Autodesk Fusion 360 part; units mm, degrees
(part 12 of 18)
  arc A1395 (119.7972, -42.2017) -> (118.5972, -42.2017) centre (119.1972, -42.2017) ccw
  arc A1396 (119.7972, -42.2017) -> (118.5972, -42.2017) centre (119.1972, -42.2017) ccw
  arc A1397 (118.5972, -42.2017) -> (119.7972, -42.2017) centre (119.1972, -42.2017) ccw
  arc A1398 (118.5972, -42.2017) -> (119.7972, -42.2017) centre (119.1972, -42.2017) ccw
  arc A1399 (119.7972, -42.2017) -> (118.5972, -42.2017) centre (119.1972, -42.2017) ccw
  arc A1400 (116.2972, -44.4557) -> (115.0972, -44.4557) centre (115.6972, -44.4557) ccw
  arc A1401 (115.0972, -44.4557) -> (116.2972, -44.4557) centre (115.6972, -44.4557) ccw
  arc A1402 (116.2972, -44.4557) -> (115.0972, -44.4557) centre (115.6972, -44.4557) ccw
  arc A1403 (115.0972, -44.4557) -> (116.2972, -44.4557) centre (115.6972, -44.4557) ccw
  arc A1404 (116.2972, -44.4557) -> (115.0972, -44.4557) centre (115.6972, -44.4557) ccw
  arc A1405 (115.0972, -44.4557) -> (116.2972, -44.4557) centre (115.6972, -44.4557) ccw
  arc A1406 (100.7472, -23.1516) -> (99.5472, -23.1516) centre (100.1472, -23.1516) ccw
  arc A1407 (99.5472, -23.1516) -> (100.7472, -23.1516) centre (100.1472, -23.1516) ccw
  arc A1408 (100.7472, -23.1516) -> (99.5472, -23.1516) centre (100.1472, -23.1516) ccw
  arc A1409 (99.5472, -23.1516) -> (100.7472, -23.1516) centre (100.1472, -23.1516) ccw
  arc A1410 (99.5472, -23.1516) -> (100.7472, -23.1516) centre (100.1472, -23.1516) ccw
  arc A1411 (100.7472, -23.1516) -> (99.5472, -23.1516) centre (100.1472, -23.1516) ccw
  arc A1412 (97.2472, -25.4057) -> (96.0472, -25.4057) centre (96.6472, -25.4057) ccw
  arc A1413 (96.0472, -25.4057) -> (97.2472, -25.4057) centre (96.6472, -25.4057) ccw
  arc A1414 (97.2472, -25.4057) -> (96.0472, -25.4057) centre (96.6472, -25.4057) ccw
  arc A1415 (96.0472, -25.4057) -> (97.2472, -25.4057) centre (96.6472, -25.4057) ccw
  arc A1416 (97.2472, -25.4057) -> (96.0472, -25.4057) centre (96.6472, -25.4057) ccw
  arc A1417 (96.0472, -25.4057) -> (97.2472, -25.4057) centre (96.6472, -25.4057) ccw
  arc A1418 (100.7472, -42.2017) -> (99.5472, -42.2017) centre (100.1472, -42.2017) ccw
  arc A1419 (99.5472, -42.2017) -> (100.7472, -42.2017) centre (100.1472, -42.2017) ccw
  arc A1420 (100.7472, -42.2017) -> (99.5472, -42.2017) centre (100.1472, -42.2017) ccw
  arc A1421 (99.5472, -42.2017) -> (100.7472, -42.2017) centre (100.1472, -42.2017) ccw
  arc A1422 (100.7472, -42.2017) -> (99.5472, -42.2017) centre (100.1472, -42.2017) ccw
  arc A1423 (99.5472, -42.2017) -> (100.7472, -42.2017) centre (100.1472, -42.2017) ccw
  arc A1424 (97.2472, -44.4557) -> (96.0472, -44.4557) centre (96.6472, -44.4557) ccw
  arc A1425 (96.0472, -44.4557) -> (97.2472, -44.4557) centre (96.6472, -44.4557) ccw
  arc A1426 (96.0472, -44.4557) -> (97.2472, -44.4557) centre (96.6472, -44.4557) ccw
  arc A1427 (97.2472, -44.4557) -> (96.0472, -44.4557) centre (96.6472, -44.4557) ccw
  arc A1428 (96.0472, -44.4557) -> (97.2472, -44.4557) centre (96.6472, -44.4557) ccw
  arc A1429 (97.2472, -44.4557) -> (96.0472, -44.4557) centre (96.6472, -44.4557) ccw
  arc A1430 (100.7472, -80.3272) -> (99.5472, -80.3272) centre (100.1472, -80.3272) ccw
  arc A1431 (99.5472, -80.3272) -> (100.7472, -80.3272) centre (100.1472, -80.3272) ccw
  arc A1432 (100.7472, -80.3272) -> (99.5472, -80.3272) centre (100.1472, -80.3272) ccw
  arc A1433 (99.5472, -80.3272) -> (100.7472, -80.3272) centre (100.1472, -80.3272) ccw
  arc A1434 (99.5472, -80.3272) -> (100.7472, -80.3272) centre (100.1472, -80.3272) ccw
  arc A1435 (100.7472, -80.3272) -> (99.5472, -80.3272) centre (100.1472, -80.3272) ccw
  arc A1436 (97.2472, -82.5812) -> (96.0472, -82.5812) centre (96.6472, -82.5812) ccw
  arc A1437 (96.0472, -82.5812) -> (97.2472, -82.5812) centre (96.6472, -82.5812) ccw
  arc A1438 (97.2472, -82.5812) -> (96.0472, -82.5812) centre (96.6472, -82.5812) ccw
  arc A1439 (96.0472, -82.5812) -> (97.2472, -82.5812) centre (96.6472, -82.5812) ccw
  arc A1440 (97.2472, -82.5812) -> (96.0472, -82.5812) centre (96.6472, -82.5812) ccw
  arc A1441 (96.0472, -82.5812) -> (97.2472, -82.5812) centre (96.6472, -82.5812) ccw
  arc A1442 (99.5472, -61.2644) -> (100.7472, -61.2644) centre (100.1472, -61.2644) ccw
  arc A1443 (100.7472, -61.2644) -> (99.5472, -61.2644) centre (100.1472, -61.2644) ccw
  arc A1444 (100.7472, -61.2644) -> (99.5472, -61.2644) centre (100.1472, -61.2644) ccw
  arc A1445 (99.5472, -61.2644) -> (100.7472, -61.2644) centre (100.1472, -61.2644) ccw
  arc A1446 (99.5472, -61.2644) -> (100.7472, -61.2644) centre (100.1472, -61.2644) ccw
  arc A1447 (100.7472, -61.2644) -> (99.5472, -61.2644) centre (100.1472, -61.2644) ccw
  arc A1448 (96.0472, -63.5184) -> (97.2472, -63.5184) centre (96.6472, -63.5184) ccw
  arc A1449 (97.2472, -63.5184) -> (96.0472, -63.5184) centre (96.6472, -63.5184) ccw
  arc A1450 (97.2472, -63.5184) -> (96.0472, -63.5184) centre (96.6472, -63.5184) ccw
  arc A1451 (96.0472, -63.5184) -> (97.2472, -63.5184) centre (96.6472, -63.5184) ccw
  arc A1452 (97.2472, -63.5184) -> (96.0472, -63.5184) centre (96.6472, -63.5184) ccw
  arc A1453 (96.0472, -63.5184) -> (97.2472, -63.5184) centre (96.6472, -63.5184) ccw
  arc A1454 (194.7974, -80.3272) -> (195.9974, -80.3272) centre (195.3974, -80.3272) ccw
  arc A1455 (195.9974, -80.3272) -> (194.7974, -80.3272) centre (195.3974, -80.3272) ccw
  arc A1456 (194.7974, -80.3272) -> (195.9974, -80.3272) centre (195.3974, -80.3272) ccw
  arc A1457 (195.9974, -80.3272) -> (194.7974, -80.3272) centre (195.3974, -80.3272) ccw
  arc A1458 (194.7974, -80.3272) -> (195.9974, -80.3272) centre (195.3974, -80.3272) ccw
  arc A1459 (195.9974, -80.3272) -> (194.7974, -80.3272) centre (195.3974, -80.3272) ccw
  arc A1460 (192.4974, -82.5812) -> (191.2974, -82.5812) centre (191.8974, -82.5812) ccw
  arc A1461 (191.2974, -82.5812) -> (192.4974, -82.5812) centre (191.8974, -82.5812) ccw
  arc A1462 (191.2974, -82.5812) -> (192.4974, -82.5812) centre (191.8974, -82.5812) ccw
  arc A1463 (192.4974, -82.5812) -> (191.2974, -82.5812) centre (191.8974, -82.5812) ccw
  arc A1464 (192.4974, -82.5812) -> (191.2974, -82.5812) centre (191.8974, -82.5812) ccw
  arc A1465 (191.2974, -82.5812) -> (192.4974, -82.5812) centre (191.8974, -82.5812) ccw
  arc A1466 (195.9974, -23.1516) -> (194.7974, -23.1516) centre (195.3974, -23.1516) ccw
  arc A1467 (194.7974, -23.1516) -> (195.9974, -23.1516) centre (195.3974, -23.1516) ccw
  arc A1468 (194.7974, -23.1516) -> (195.9974, -23.1516) centre (195.3974, -23.1516) ccw
  arc A1469 (195.9974, -23.1516) -> (194.7974, -23.1516) centre (195.3974, -23.1516) ccw
  arc A1470 (195.9974, -23.1516) -> (194.7974, -23.1516) centre (195.3974, -23.1516) ccw
  arc A1471 (194.7974, -23.1516) -> (195.9974, -23.1516) centre (195.3974, -23.1516) ccw
  arc A1472 (192.4974, -25.4057) -> (191.2974, -25.4057) centre (191.8974, -25.4057) ccw
  arc A1473 (191.2974, -25.4057) -> (192.4974, -25.4057) centre (191.8974, -25.4057) ccw
  arc A1474 (191.2974, -25.4057) -> (192.4974, -25.4057) centre (191.8974, -25.4057) ccw
  arc A1475 (192.4974, -25.4057) -> (191.2974, -25.4057) centre (191.8974, -25.4057) ccw
  arc A1476 (192.4974, -25.4057) -> (191.2974, -25.4057) centre (191.8974, -25.4057) ccw
  arc A1477 (191.2974, -25.4057) -> (192.4974, -25.4057) centre (191.8974, -25.4057) ccw
  arc A1478 (81.6972, -80.3272) -> (80.4972, -80.3272) centre (81.0972, -80.3272) ccw
  arc A1479 (80.4972, -80.3272) -> (81.6972, -80.3272) centre (81.0972, -80.3272) ccw
  arc A1480 (81.6972, -80.3272) -> (80.4972, -80.3272) centre (81.0972, -80.3272) ccw
  arc A1481 (80.4972, -80.3272) -> (81.6972, -80.3272) centre (81.0972, -80.3272) ccw
  arc A1482 (80.4972, -80.3272) -> (81.6972, -80.3272) centre (81.0972, -80.3272) ccw
  arc A1483 (81.6972, -80.3272) -> (80.4972, -80.3272) centre (81.0972, -80.3272) ccw
  arc A1484 (76.9972, -82.5812) -> (78.1972, -82.5812) centre (77.5972, -82.5812) ccw
  arc A1485 (78.1972, -82.5812) -> (76.9972, -82.5812) centre (77.5972, -82.5812) ccw
  arc A1486 (76.9972, -82.5812) -> (78.1972, -82.5812) centre (77.5972, -82.5812) ccw
  arc A1487 (78.1972, -82.5812) -> (76.9972, -82.5812) centre (77.5972, -82.5812) ccw
  arc A1488 (78.1972, -82.5812) -> (76.9972, -82.5812) centre (77.5972, -82.5812) ccw
  arc A1489 (76.9972, -82.5812) -> (78.1972, -82.5812) centre (77.5972, -82.5812) ccw
  arc A1490 (81.6972, -42.2017) -> (80.4972, -42.2017) centre (81.0972, -42.2017) ccw
  arc A1491 (80.4972, -42.2017) -> (81.6972, -42.2017) centre (81.0972, -42.2017) ccw
  arc A1492 (81.6972, -42.2017) -> (80.4972, -42.2017) centre (81.0972, -42.2017) ccw
  arc A1493 (80.4972, -42.2017) -> (81.6972, -42.2017) centre (81.0972, -42.2017) ccw
  arc A1494 (81.6972, -42.2017) -> (80.4972, -42.2017) centre (81.0972, -42.2017) ccw
  arc A1495 (80.4972, -42.2017) -> (81.6972, -42.2017) centre (81.0972, -42.2017) ccw
  arc A1496 (78.1972, -44.4557) -> (76.9972, -44.4557) centre (77.5972, -44.4557) ccw
  arc A1497 (76.9972, -44.4557) -> (78.1972, -44.4557) centre (77.5972, -44.4557) ccw
  arc A1498 (76.9972, -44.4557) -> (78.1972, -44.4557) centre (77.5972, -44.4557) ccw
  arc A1499 (78.1972, -44.4557) -> (76.9972, -44.4557) centre (77.5972, -44.4557) ccw
  arc A1500 (78.1972, -44.4557) -> (76.9972, -44.4557) centre (77.5972, -44.4557) ccw
  arc A1501 (76.9972, -44.4557) -> (78.1972, -44.4557) centre (77.5972, -44.4557) ccw
  arc A1502 (80.4972, -23.1516) -> (81.6972, -23.1516) centre (81.0972, -23.1516) ccw
  arc A1503 (81.6972, -23.1516) -> (80.4972, -23.1516) centre (81.0972, -23.1516) ccw
  arc A1504 (80.4972, -23.1516) -> (81.6972, -23.1516) centre (81.0972, -23.1516) ccw
  arc A1505 (81.6972, -23.1516) -> (80.4972, -23.1516) centre (81.0972, -23.1516) ccw
  arc A1506 (81.6972, -23.1516) -> (80.4972, -23.1516) centre (81.0972, -23.1516) ccw
  arc A1507 (80.4972, -23.1516) -> (81.6972, -23.1516) centre (81.0972, -23.1516) ccw
  arc A1508 (78.1972, -25.4057) -> (76.9972, -25.4057) centre (77.5972, -25.4057) ccw
  arc A1509 (76.9972, -25.4057) -> (78.1972, -25.4057) centre (77.5972, -25.4057) ccw
  arc A1510 (76.9972, -25.4057) -> (78.1972, -25.4057) centre (77.5972, -25.4057) ccw
  arc A1511 (78.1972, -25.4057) -> (76.9972, -25.4057) centre (77.5972, -25.4057) ccw
  arc A1512 (76.9972, -25.4057) -> (78.1972, -25.4057) centre (77.5972, -25.4057) ccw
  arc A1513 (78.1972, -25.4057) -> (76.9972, -25.4057) centre (77.5972, -25.4057) ccw
  arc A1514 (80.4972, -61.2644) -> (81.6972, -61.2644) centre (81.0972, -61.2644) ccw
  arc A1515 (81.6972, -61.2644) -> (80.4972, -61.2644) centre (81.0972, -61.2644) ccw
  arc A1516 (81.6972, -61.2644) -> (80.4972, -61.2644) centre (81.0972, -61.2644) ccw
  arc A1517 (80.4972, -61.2644) -> (81.6972, -61.2644) centre (81.0972, -61.2644) ccw
  arc A1518 (81.6972, -61.2644) -> (80.4972, -61.2644) centre (81.0972, -61.2644) ccw
  arc A1519 (80.4972, -61.2644) -> (81.6972, -61.2644) centre (81.0972, -61.2644) ccw
  arc A1520 (76.9972, -63.5184) -> (78.1972, -63.5184) centre (77.5972, -63.5184) ccw
  arc A1521 (78.1972, -63.5184) -> (76.9972, -63.5184) centre (77.5972, -63.5184) ccw
  arc A1522 (78.1972, -63.5184) -> (76.9972, -63.5184) centre (77.5972, -63.5184) ccw
  arc A1523 (76.9972, -63.5184) -> (78.1972, -63.5184) centre (77.5972, -63.5184) ccw
  arc A1524 (78.1972, -63.5184) -> (76.9972, -63.5184) centre (77.5972, -63.5184) ccw
  arc A1525 (76.9972, -63.5184) -> (78.1972, -63.5184) centre (77.5972, -63.5184) ccw
  arc A1526 (61.4471, -80.3272) -> (62.6471, -80.3272) centre (62.0471, -80.3272) ccw
  arc A1527 (62.6471, -80.3272) -> (61.4471, -80.3272) centre (62.0471, -80.3272) ccw
  arc A1528 (61.4471, -80.3272) -> (62.6471, -80.3272) centre (62.0471, -80.3272) ccw
  arc A1529 (62.6471, -80.3272) -> (61.4471, -80.3272) centre (62.0471, -80.3272) ccw
  arc A1530 (61.4471, -80.3272) -> (62.6471, -80.3272) centre (62.0471, -80.3272) ccw
  arc A1531 (62.6471, -80.3272) -> (61.4471, -80.3272) centre (62.0471, -80.3272) ccw
  arc A1532 (59.1471, -82.5812) -> (57.9471, -82.5812) centre (58.5471, -82.5812) ccw
  arc A1533 (57.9471, -82.5812) -> (59.1471, -82.5812) centre (58.5471, -82.5812) ccw
  arc A1534 (57.9471, -82.5812) -> (59.1471, -82.5812) centre (58.5471, -82.5812) ccw
  arc A1535 (59.1471, -82.5812) -> (57.9471, -82.5812) centre (58.5471, -82.5812) ccw
  arc A1536 (57.9471, -82.5812) -> (59.1471, -82.5812) centre (58.5471, -82.5812) ccw
  arc A1537 (59.1471, -82.5812) -> (57.9471, -82.5812) centre (58.5471, -82.5812) ccw
  arc A1538 (61.4471, -61.2644) -> (62.6471, -61.2644) centre (62.0471, -61.2644) ccw
  arc A1539 (62.6471, -61.2644) -> (61.4471, -61.2644) centre (62.0471, -61.2644) ccw
  arc A1540 (62.6471, -61.2644) -> (61.4471, -61.2644) centre (62.0471, -61.2644) ccw
  arc A1541 (61.4471, -61.2644) -> (62.6471, -61.2644) centre (62.0471, -61.2644) ccw
  arc A1542 (62.6471, -61.2644) -> (61.4471, -61.2644) centre (62.0471, -61.2644) ccw
  arc A1543 (61.4471, -61.2644) -> (62.6471, -61.2644) centre (62.0471, -61.2644) ccw
  arc A1544 (57.9471, -63.5184) -> (59.1471, -63.5184) centre (58.5471, -63.5184) ccw
  arc A1545 (59.1471, -63.5184) -> (57.9471, -63.5184) centre (58.5471, -63.5184) ccw
  arc A1546 (59.1471, -63.5184) -> (57.9471, -63.5184) centre (58.5471, -63.5184) ccw
  arc A1547 (57.9471, -63.5184) -> (59.1471, -63.5184) centre (58.5471, -63.5184) ccw
  arc A1548 (57.9471, -63.5184) -> (59.1471, -63.5184) centre (58.5471, -63.5184) ccw
  arc A1549 (59.1471, -63.5184) -> (57.9471, -63.5184) centre (58.5471, -63.5184) ccw
  arc A1550 (61.4471, -42.2017) -> (62.6471, -42.2017) centre (62.0471, -42.2017) ccw
  arc A1551 (62.6471, -42.2017) -> (61.4471, -42.2017) centre (62.0471, -42.2017) ccw
  arc A1552 (61.4471, -42.2017) -> (62.6471, -42.2017) centre (62.0471, -42.2017) ccw
  arc A1553 (62.6471, -42.2017) -> (61.4471, -42.2017) centre (62.0471, -42.2017) ccw
  arc A1554 (61.4471, -42.2017) -> (62.6471, -42.2017) centre (62.0471, -42.2017) ccw
  arc A1555 (62.6471, -42.2017) -> (61.4471, -42.2017) centre (62.0471, -42.2017) ccw
  arc A1556 (59.1471, -44.4557) -> (57.9471, -44.4557) centre (58.5471, -44.4557) ccw
  arc A1557 (57.9471, -44.4557) -> (59.1471, -44.4557) centre (58.5471, -44.4557) ccw
  arc A1558 (57.9471, -44.4557) -> (59.1471, -44.4557) centre (58.5471, -44.4557) ccw
  arc A1559 (59.1471, -44.4557) -> (57.9471, -44.4557) centre (58.5471, -44.4557) ccw
  arc A1560 (59.1471, -44.4557) -> (57.9471, -44.4557) centre (58.5471, -44.4557) ccw
  arc A1561 (57.9471, -44.4557) -> (59.1471, -44.4557) centre (58.5471, -44.4557) ccw
  arc A1562 (42.3971, -61.2644) -> (43.5971, -61.2644) centre (42.9971, -61.2644) ccw
  arc A1563 (43.5971, -61.2644) -> (42.3971, -61.2644) centre (42.9971, -61.2644) ccw
  arc A1564 (43.5971, -61.2644) -> (42.3971, -61.2644) centre (42.9971, -61.2644) ccw
  arc A1565 (42.3971, -61.2644) -> (43.5971, -61.2644) centre (42.9971, -61.2644) ccw
  arc A1566 (43.5971, -61.2644) -> (42.3971, -61.2644) centre (42.9971, -61.2644) ccw
  arc A1567 (42.3971, -61.2644) -> (43.5971, -61.2644) centre (42.9971, -61.2644) ccw
  arc A1568 (40.0971, -63.5184) -> (38.8971, -63.5184) centre (39.4971, -63.5184) ccw
  arc A1569 (38.8971, -63.5184) -> (40.0971, -63.5184) centre (39.4971, -63.5184) ccw
  arc A1570 (40.0971, -63.5184) -> (38.8971, -63.5184) centre (39.4971, -63.5184) ccw
  arc A1571 (38.8971, -63.5184) -> (40.0971, -63.5184) centre (39.4971, -63.5184) ccw
  arc A1572 (40.0971, -63.5184) -> (38.8971, -63.5184) centre (39.4971, -63.5184) ccw
  arc A1573 (38.8971, -63.5184) -> (40.0971, -63.5184) centre (39.4971, -63.5184) ccw
  arc A1574 (42.3971, -80.3272) -> (43.5971, -80.3272) centre (42.9971, -80.3272) ccw
  arc A1575 (43.5971, -80.3272) -> (42.3971, -80.3272) centre (42.9971, -80.3272) ccw
  arc A1576 (43.5971, -80.3272) -> (42.3971, -80.3272) centre (42.9971, -80.3272) ccw
  arc A1577 (42.3971, -80.3272) -> (43.5971, -80.3272) centre (42.9971, -80.3272) ccw
  arc A1578 (42.3971, -80.3272) -> (43.5971, -80.3272) centre (42.9971, -80.3272) ccw
  arc A1579 (43.5971, -80.3272) -> (42.3971, -80.3272) centre (42.9971, -80.3272) ccw
  arc A1580 (40.0971, -82.5812) -> (38.8971, -82.5812) centre (39.4971, -82.5812) ccw
  arc A1581 (38.8971, -82.5812) -> (40.0971, -82.5812) centre (39.4971, -82.5812) ccw
  arc A1582 (38.8971, -82.5812) -> (40.0971, -82.5812) centre (39.4971, -82.5812) ccw
  arc A1583 (40.0971, -82.5812) -> (38.8971, -82.5812) centre (39.4971, -82.5812) ccw
  arc A1584 (40.0971, -82.5812) -> (38.8971, -82.5812) centre (39.4971, -82.5812) ccw
  arc A1585 (38.8971, -82.5812) -> (40.0971, -82.5812) centre (39.4971, -82.5812) ccw
  arc A1586 (24.547, -80.3272) -> (23.347, -80.3272) centre (23.947, -80.3272) ccw
  arc A1587 (23.347, -80.3272) -> (24.547, -80.3272) centre (23.947, -80.3272) ccw
  arc A1588 (23.347, -80.3272) -> (24.547, -80.3272) centre (23.947, -80.3272) ccw
  arc A1589 (24.547, -80.3272) -> (23.347, -80.3272) centre (23.947, -80.3272) ccw
  arc A1590 (23.347, -80.3272) -> (24.547, -80.3272) centre (23.947, -80.3272) ccw
  arc A1591 (24.547, -80.3272) -> (23.347, -80.3272) centre (23.947, -80.3272) ccw
  arc A1592 (21.047, -82.5812) -> (19.847, -82.5812) centre (20.447, -82.5812) ccw
  arc A1593 (19.847, -82.5812) -> (21.047, -82.5812) centre (20.447, -82.5812) ccw
  arc A1594 (19.847, -82.5812) -> (21.047, -82.5812) centre (20.447, -82.5812) ccw
  arc A1595 (21.047, -82.5812) -> (19.847, -82.5812) centre (20.447, -82.5812) ccw
  arc A1596 (19.847, -82.5812) -> (21.047, -82.5812) centre (20.447, -82.5812) ccw
  arc A1597 (21.047, -82.5812) -> (19.847, -82.5812) centre (20.447, -82.5812) ccw
  arc A1598 (5.497, -80.3272) -> (4.297, -80.3272) centre (4.897, -80.3272) ccw
  arc A1599 (4.297, -80.3272) -> (5.497, -80.3272) centre (4.897, -80.3272) ccw
  arc A1600 (4.297, -80.3272) -> (5.497, -80.3272) centre (4.897, -80.3272) ccw
  arc A1601 (5.497, -80.3272) -> (4.297, -80.3272) centre (4.897, -80.3272) ccw
  arc A1602 (5.497, -80.3272) -> (4.297, -80.3272) centre (4.897, -80.3272) ccw
  arc A1603 (4.297, -80.3272) -> (5.497, -80.3272) centre (4.897, -80.3272) ccw
  arc A1604 (1.997, -82.5812) -> (0.797, -82.5812) centre (1.397, -82.5812) ccw
  arc A1605 (0.797, -82.5812) -> (1.997, -82.5812) centre (1.397, -82.5812) ccw
  arc A1606 (0.797, -82.5812) -> (1.997, -82.5812) centre (1.397, -82.5812) ccw
  arc A1607 (1.997, -82.5812) -> (0.797, -82.5812) centre (1.397, -82.5812) ccw
  arc A1608 (0.797, -82.5812) -> (1.997, -82.5812) centre (1.397, -82.5812) ccw
  arc A1609 (1.997, -82.5812) -> (0.797, -82.5812) centre (1.397, -82.5812) ccw
  arc A1610 (61.4471, -23.1516) -> (62.6471, -23.1516) centre (62.0471, -23.1516) ccw
  arc A1611 (62.6471, -23.1516) -> (61.4471, -23.1516) centre (62.0471, -23.1516) ccw
  arc A1612 (62.6471, -23.1516) -> (61.4471, -23.1516) centre (62.0471, -23.1516) ccw
  arc A1613 (61.4471, -23.1516) -> (62.6471, -23.1516) centre (62.0471, -23.1516) ccw
  arc A1614 (61.4471, -23.1516) -> (62.6471, -23.1516) centre (62.0471, -23.1516) ccw
  arc A1615 (62.6471, -23.1516) -> (61.4471, -23.1516) centre (62.0471, -23.1516) ccw
  arc A1616 (59.1471, -25.4057) -> (57.9471, -25.4057) centre (58.5471, -25.4057) ccw
  arc A1617 (57.9471, -25.4057) -> (59.1471, -25.4057) centre (58.5471, -25.4057) ccw
  arc A1618 (57.9471, -25.4057) -> (59.1471, -25.4057) centre (58.5471, -25.4057) ccw
  arc A1619 (59.1471, -25.4057) -> (57.9471, -25.4057) centre (58.5471, -25.4057) ccw
  arc A1620 (57.9471, -25.4057) -> (59.1471, -25.4057) centre (58.5471, -25.4057) ccw
  arc A1621 (59.1471, -25.4057) -> (57.9471, -25.4057) centre (58.5471, -25.4057) ccw
  arc A1622 (42.3971, -42.2017) -> (43.5971, -42.2017) centre (42.9971, -42.2017) ccw
  arc A1623 (43.5971, -42.2017) -> (42.3971, -42.2017) centre (42.9971, -42.2017) ccw
  arc A1624 (43.5971, -42.2017) -> (42.3971, -42.2017) centre (42.9971, -42.2017) ccw
  arc A1625 (42.3971, -42.2017) -> (43.5971, -42.2017) centre (42.9971, -42.2017) ccw
  arc A1626 (43.5971, -42.2017) -> (42.3971, -42.2017) centre (42.9971, -42.2017) ccw
  arc A1627 (42.3971, -42.2017) -> (43.5971, -42.2017) centre (42.9971, -42.2017) ccw
  arc A1628 (40.0971, -44.4557) -> (38.8971, -44.4557) centre (39.4971, -44.4557) ccw
  arc A1629 (38.8971, -44.4557) -> (40.0971, -44.4557) centre (39.4971, -44.4557) ccw
  arc A1630 (38.8971, -44.4557) -> (40.0971, -44.4557) centre (39.4971, -44.4557) ccw
  arc A1631 (40.0971, -44.4557) -> (38.8971, -44.4557) centre (39.4971, -44.4557) ccw
  arc A1632 (38.8971, -44.4557) -> (40.0971, -44.4557) centre (39.4971, -44.4557) ccw
  arc A1633 (40.0971, -44.4557) -> (38.8971, -44.4557) centre (39.4971, -44.4557) ccw
  arc A1634 (43.5971, -23.1516) -> (42.3971, -23.1516) centre (42.9971, -23.1516) ccw
  arc A1635 (42.3971, -23.1516) -> (43.5971, -23.1516) centre (42.9971, -23.1516) ccw
  arc A1636 (42.3971, -23.1516) -> (43.5971, -23.1516) centre (42.9971, -23.1516) ccw
  arc A1637 (43.5971, -23.1516) -> (42.3971, -23.1516) centre (42.9971, -23.1516) ccw
  arc A1638 (43.5971, -23.1516) -> (42.3971, -23.1516) centre (42.9971, -23.1516) ccw
  arc A1639 (42.3971, -23.1516) -> (43.5971, -23.1516) centre (42.9971, -23.1516) ccw
  arc A1640 (38.8971, -25.4057) -> (40.0971, -25.4057) centre (39.4971, -25.4057) ccw
  arc A1641 (40.0971, -25.4057) -> (38.8971, -25.4057) centre (39.4971, -25.4057) ccw
  arc A1642 (40.0971, -25.4057) -> (38.8971, -25.4057) centre (39.4971, -25.4057) ccw
  arc A1643 (38.8971, -25.4057) -> (40.0971, -25.4057) centre (39.4971, -25.4057) ccw
  arc A1644 (38.8971, -25.4057) -> (40.0971, -25.4057) centre (39.4971, -25.4057) ccw
  arc A1645 (40.0971, -25.4057) -> (38.8971, -25.4057) centre (39.4971, -25.4057) ccw
  arc A1646 (23.347, -23.1516) -> (24.547, -23.1516) centre (23.947, -23.1516) ccw
  arc A1647 (24.547, -23.1516) -> (23.347, -23.1516) centre (23.947, -23.1516) ccw
  arc A1648 (23.347, -23.1516) -> (24.547, -23.1516) centre (23.947, -23.1516) ccw
  arc A1649 (24.547, -23.1516) -> (23.347, -23.1516) centre (23.947, -23.1516) ccw
  arc A1650 (23.347, -23.1516) -> (24.547, -23.1516) centre (23.947, -23.1516) ccw
  arc A1651 (24.547, -23.1516) -> (23.347, -23.1516) centre (23.947, -23.1516) ccw
  arc A1652 (21.047, -25.4057) -> (19.847, -25.4057) centre (20.447, -25.4057) ccw
  arc A1653 (19.847, -25.4057) -> (21.047, -25.4057) centre (20.447, -25.4057) ccw
  arc A1654 (19.847, -25.4057) -> (21.047, -25.4057) centre (20.447, -25.4057) ccw
  arc A1655 (21.047, -25.4057) -> (19.847, -25.4057) centre (20.447, -25.4057) ccw
  arc A1656 (19.847, -25.4057) -> (21.047, -25.4057) centre (20.447, -25.4057) ccw
  arc A1657 (21.047, -25.4057) -> (19.847, -25.4057) centre (20.447, -25.4057) ccw
  arc A1658 (24.547, -61.2644) -> (23.347, -61.2644) centre (23.947, -61.2644) ccw
  arc A1659 (23.347, -61.2644) -> (24.547, -61.2644) centre (23.947, -61.2644) ccw
  arc A1660 (23.347, -61.2644) -> (24.547, -61.2644) centre (23.947, -61.2644) ccw
  arc A1661 (24.547, -61.2644) -> (23.347, -61.2644) centre (23.947, -61.2644) ccw
  arc A1662 (23.347, -61.2644) -> (24.547, -61.2644) centre (23.947, -61.2644) ccw
  arc A1663 (24.547, -61.2644) -> (23.347, -61.2644) centre (23.947, -61.2644) ccw
  arc A1664 (19.847, -63.5184) -> (21.047, -63.5184) centre (20.447, -63.5184) ccw
  arc A1665 (21.047, -63.5184) -> (19.847, -63.5184) centre (20.447, -63.5184) ccw
  arc A1666 (21.047, -63.5184) -> (19.847, -63.5184) centre (20.447, -63.5184) ccw
  arc A1667 (19.847, -63.5184) -> (21.047, -63.5184) centre (20.447, -63.5184) ccw
  arc A1668 (21.047, -63.5184) -> (19.847, -63.5184) centre (20.447, -63.5184) ccw
  arc A1669 (19.847, -63.5184) -> (21.047, -63.5184) centre (20.447, -63.5184) ccw
  arc A1670 (23.347, -42.2017) -> (24.547, -42.2017) centre (23.947, -42.2017) ccw
  arc A1671 (24.547, -42.2017) -> (23.347, -42.2017) centre (23.947, -42.2017) ccw
  arc A1672 (24.547, -42.2017) -> (23.347, -42.2017) centre (23.947, -42.2017) ccw
  arc A1673 (23.347, -42.2017) -> (24.547, -42.2017) centre (23.947, -42.2017) ccw
  arc A1674 (24.547, -42.2017) -> (23.347, -42.2017) centre (23.947, -42.2017) ccw
  arc A1675 (23.347, -42.2017) -> (24.547, -42.2017) centre (23.947, -42.2017) ccw
  arc A1676 (19.847, -44.4557) -> (21.047, -44.4557) centre (20.447, -44.4557) ccw
  arc A1677 (21.047, -44.4557) -> (19.847, -44.4557) centre (20.447, -44.4557) ccw
  arc A1678 (19.847, -44.4557) -> (21.047, -44.4557) centre (20.447, -44.4557) ccw
  arc A1679 (21.047, -44.4557) -> (19.847, -44.4557) centre (20.447, -44.4557) ccw
  arc A1680 (21.047, -44.4557) -> (19.847, -44.4557) centre (20.447, -44.4557) ccw
  arc A1681 (19.847, -44.4557) -> (21.047, -44.4557) centre (20.447, -44.4557) ccw
  arc A1682 (4.297, -23.1516) -> (5.497, -23.1516) centre (4.897, -23.1516) ccw
  arc A1683 (5.497, -23.1516) -> (4.297, -23.1516) centre (4.897, -23.1516) ccw
  arc A1684 (5.497, -23.1516) -> (4.297, -23.1516) centre (4.897, -23.1516) ccw
  arc A1685 (4.297, -23.1516) -> (5.497, -23.1516) centre (4.897, -23.1516) ccw
  arc A1686 (5.497, -23.1516) -> (4.297, -23.1516) centre (4.897, -23.1516) ccw
  arc A1687 (4.297, -23.1516) -> (5.497, -23.1516) centre (4.897, -23.1516) ccw
  arc A1688 (1.997, -25.4057) -> (0.797, -25.4057) centre (1.397, -25.4057) ccw
  arc A1689 (0.797, -25.4057) -> (1.997, -25.4057) centre (1.397, -25.4057) ccw
  arc A1690 (0.797, -25.4057) -> (1.997, -25.4057) centre (1.397, -25.4057) ccw
  arc A1691 (1.997, -25.4057) -> (0.797, -25.4057) centre (1.397, -25.4057) ccw
  arc A1692 (1.997, -25.4057) -> (0.797, -25.4057) centre (1.397, -25.4057) ccw
  arc A1693 (0.797, -25.4057) -> (1.997, -25.4057) centre (1.397, -25.4057) ccw
  arc A1694 (5.497, -42.2017) -> (4.297, -42.2017) centre (4.897, -42.2017) ccw
  arc A1695 (4.297, -42.2017) -> (5.497, -42.2017) centre (4.897, -42.2017) ccw
  arc A1696 (5.497, -42.2017) -> (4.297, -42.2017) centre (4.897, -42.2017) ccw
  arc A1697 (4.297, -42.2017) -> (5.497, -42.2017) centre (4.897, -42.2017) ccw
  arc A1698 (5.497, -42.2017) -> (4.297, -42.2017) centre (4.897, -42.2017) ccw
  arc A1699 (4.297, -42.2017) -> (5.497, -42.2017) centre (4.897, -42.2017) ccw
  arc A1700 (1.997, -44.4557) -> (0.797, -44.4557) centre (1.397, -44.4557) ccw
  arc A1701 (0.797, -44.4557) -> (1.997, -44.4557) centre (1.397, -44.4557) ccw
  arc A1702 (1.997, -44.4557) -> (0.797, -44.4557) centre (1.397, -44.4557) ccw
  arc A1703 (0.797, -44.4557) -> (1.997, -44.4557) centre (1.397, -44.4557) ccw
  arc A1704 (1.997, -44.4557) -> (0.797, -44.4557) centre (1.397, -44.4557) ccw
  arc A1705 (0.797, -44.4557) -> (1.997, -44.4557) centre (1.397, -44.4557) ccw
  arc A1706 (5.497, -61.2644) -> (4.297, -61.2644) centre (4.897, -61.2644) ccw
  arc A1707 (4.297, -61.2644) -> (5.497, -61.2644) centre (4.897, -61.2644) ccw
  arc A1708 (4.297, -61.2644) -> (5.497, -61.2644) centre (4.897, -61.2644) ccw
  arc A1709 (5.497, -61.2644) -> (4.297, -61.2644) centre (4.897, -61.2644) ccw
  arc A1710 (4.297, -61.2644) -> (5.497, -61.2644) centre (4.897, -61.2644) ccw
  arc A1711 (5.497, -61.2644) -> (4.297, -61.2644) centre (4.897, -61.2644) ccw
  arc A1712 (0.797, -63.5184) -> (1.997, -63.5184) centre (1.397, -63.5184) ccw
  arc A1713 (1.997, -63.5184) -> (0.797, -63.5184) centre (1.397, -63.5184) ccw
  arc A1714 (1.997, -63.5184) -> (0.797, -63.5184) centre (1.397, -63.5184) ccw
  arc A1715 (0.797, -63.5184) -> (1.997, -63.5184) centre (1.397, -63.5184) ccw
  arc A1716 (1.997, -63.5184) -> (0.797, -63.5184) centre (1.397, -63.5184) ccw
  arc A1717 (0.797, -63.5184) -> (1.997, -63.5184) centre (1.397, -63.5184) ccw
  arc A1718 (215.0474, -61.2644) -> (213.8474, -61.2644) centre (214.4474, -61.2644) ccw
  arc A1719 (213.8474, -61.2644) -> (215.0474, -61.2644) centre (214.4474, -61.2644) ccw
  arc A1720 (215.0474, -61.2644) -> (213.8474, -61.2644) centre (214.4474, -61.2644) ccw
  arc A1721 (213.8474, -61.2644) -> (215.0474, -61.2644) centre (214.4474, -61.2644) ccw
  arc A1722 (215.0474, -61.2644) -> (213.8474, -61.2644) centre (214.4474, -61.2644) ccw
  arc A1723 (213.8474, -61.2644) -> (215.0474, -61.2644) centre (214.4474, -61.2644) ccw
  arc A1724 (211.5474, -63.5184) -> (210.3474, -63.5184) centre (210.9474, -63.5184) ccw
  arc A1725 (210.3474, -63.5184) -> (211.5474, -63.5184) centre (210.9474, -63.5184) ccw
  arc A1726 (210.3474, -63.5184) -> (211.5474, -63.5184) centre (210.9474, -63.5184) ccw
  arc A1727 (211.5474, -63.5184) -> (210.3474, -63.5184) centre (210.9474, -63.5184) ccw
  arc A1728 (210.3474, -63.5184) -> (211.5474, -63.5184) centre (210.9474, -63.5184) ccw
  arc A1729 (211.5474, -63.5184) -> (210.3474, -63.5184) centre (210.9474, -63.5184) ccw
  arc A1730 (215.0474, -42.2017) -> (213.8474, -42.2017) centre (214.4474, -42.2017) ccw
  arc A1731 (213.8474, -42.2017) -> (215.0474, -42.2017) centre (214.4474, -42.2017) ccw
  arc A1732 (213.8474, -42.2017) -> (215.0474, -42.2017) centre (214.4474, -42.2017) ccw
  arc A1733 (215.0474, -42.2017) -> (213.8474, -42.2017) centre (214.4474, -42.2017) ccw
  arc A1734 (213.8474, -42.2017) -> (215.0474, -42.2017) centre (214.4474, -42.2017) ccw
  arc A1735 (215.0474, -42.2017) -> (213.8474, -42.2017) centre (214.4474, -42.2017) ccw
  arc A1736 (210.3474, -44.4557) -> (211.5474, -44.4557) centre (210.9474, -44.4557) ccw
  arc A1737 (211.5474, -44.4557) -> (210.3474, -44.4557) centre (210.9474, -44.4557) ccw
  arc A1738 (211.5474, -44.4557) -> (210.3474, -44.4557) centre (210.9474, -44.4557) ccw
  arc A1739 (210.3474, -44.4557) -> (211.5474, -44.4557) centre (210.9474, -44.4557) ccw
  arc A1740 (210.3474, -44.4557) -> (211.5474, -44.4557) centre (210.9474, -44.4557) ccw
  arc A1741 (211.5474, -44.4557) -> (210.3474, -44.4557) centre (210.9474, -44.4557) ccw
  arc A1742 (215.0474, -23.1516) -> (213.8474, -23.1516) centre (214.4474, -23.1516) ccw
  arc A1743 (213.8474, -23.1516) -> (215.0474, -23.1516) centre (214.4474, -23.1516) ccw
  arc A1744 (215.0474, -23.1516) -> (213.8474, -23.1516) centre (214.4474, -23.1516) ccw
  arc A1745 (213.8474, -23.1516) -> (215.0474, -23.1516) centre (214.4474, -23.1516) ccw
  arc A1746 (215.0474, -23.1516) -> (213.8474, -23.1516) centre (214.4474, -23.1516) ccw
  arc A1747 (213.8474, -23.1516) -> (215.0474, -23.1516) centre (214.4474, -23.1516) ccw
  arc A1748 (210.3474, -25.4057) -> (211.5474, -25.4057) centre (210.9474, -25.4057) ccw
  arc A1749 (211.5474, -25.4057) -> (210.3474, -25.4057) centre (210.9474, -25.4057) ccw
  arc A1750 (210.3474, -25.4057) -> (211.5474, -25.4057) centre (210.9474, -25.4057) ccw
  arc A1751 (211.5474, -25.4057) -> (210.3474, -25.4057) centre (210.9474, -25.4057) ccw
  arc A1752 (211.5474, -25.4057) -> (210.3474, -25.4057) centre (210.9474, -25.4057) ccw
  arc A1753 (210.3474, -25.4057) -> (211.5474, -25.4057) centre (210.9474, -25.4057) ccw
  arc A1754 (213.8474, -80.3272) -> (215.0474, -80.3272) centre (214.4474, -80.3272) ccw
  arc A1755 (215.0474, -80.3272) -> (213.8474, -80.3272) centre (214.4474, -80.3272) ccw
  arc A1756 (213.8474, -80.3272) -> (215.0474, -80.3272) centre (214.4474, -80.3272) ccw
  arc A1757 (215.0474, -80.3272) -> (213.8474, -80.3272) centre (214.4474, -80.3272) ccw
  arc A1758 (213.8474, -80.3272) -> (215.0474, -80.3272) centre (214.4474, -80.3272) ccw
  arc A1759 (215.0474, -80.3272) -> (213.8474, -80.3272) centre (214.4474, -80.3272) ccw
  arc A1760 (211.5474, -82.5812) -> (210.3474, -82.5812) centre (210.9474, -82.5812) ccw
  arc A1761 (210.3474, -82.5812) -> (211.5474, -82.5812) centre (210.9474, -82.5812) ccw
  arc A1762 (210.3474, -82.5812) -> (211.5474, -82.5812) centre (210.9474, -82.5812) ccw
  arc A1763 (211.5474, -82.5812) -> (210.3474, -82.5812) centre (210.9474, -82.5812) ccw
  arc A1764 (210.3474, -82.5812) -> (211.5474, -82.5812) centre (210.9474, -82.5812) ccw
  arc A1765 (211.5474, -82.5812) -> (210.3474, -82.5812) centre (210.9474, -82.5812) ccw
  arc A1766 (194.7974, -42.2017) -> (195.9974, -42.2017) centre (195.3974, -42.2017) ccw
  arc A1767 (195.9974, -42.2017) -> (194.7974, -42.2017) centre (195.3974, -42.2017) ccw
  arc A1768 (195.9974, -42.2017) -> (194.7974, -42.2017) centre (195.3974, -42.2017) ccw
  arc A1769 (194.7974, -42.2017) -> (195.9974, -42.2017) centre (195.3974, -42.2017) ccw
  arc A1770 (195.9974, -42.2017) -> (194.7974, -42.2017) centre (195.3974, -42.2017) ccw
  arc A1771 (194.7974, -42.2017) -> (195.9974, -42.2017) centre (195.3974, -42.2017) ccw
  arc A1772 (191.2974, -44.4557) -> (192.4974, -44.4557) centre (191.8974, -44.4557) ccw
  arc A1773 (192.4974, -44.4557) -> (191.2974, -44.4557) centre (191.8974, -44.4557) ccw
  arc A1774 (192.4974, -44.4557) -> (191.2974, -44.4557) centre (191.8974, -44.4557) ccw
  arc A1775 (191.2974, -44.4557) -> (192.4974, -44.4557) centre (191.8974, -44.4557) ccw
  arc A1776 (192.4974, -44.4557) -> (191.2974, -44.4557) centre (191.8974, -44.4557) ccw
  arc A1777 (191.2974, -44.4557) -> (192.4974, -44.4557) centre (191.8974, -44.4557) ccw
  arc A1778 (175.1224, -4.318) -> (176.9224, -4.318) centre (176.0224, -4.318) ccw
  arc A1779 (176.9224, -4.318) -> (175.1224, -4.318) centre (176.0224, -4.318) ccw
  arc A1780 (176.9224, -4.318) -> (175.1224, -4.318) centre (176.0224, -4.318) ccw
  arc A1781 (175.1224, -4.318) -> (176.9224, -4.318) centre (176.0224, -4.318) ccw
  arc A1782 (176.9224, -4.318) -> (175.1224, -4.318) centre (176.0224, -4.318) ccw
  arc A1783 (175.1224, -4.318) -> (176.9224, -4.318) centre (176.0224, -4.318) ccw
  line L7684 (174.3823, -3.418) -> (174.3823, -5.218)
  line L7685 (172.5823, -3.418) -> (174.3823, -3.418)
  line L7686 (174.3823, -5.218) -> (172.5823, -5.218)
  line L7687 (172.5823, -5.218) -> (172.5823, -3.418)
  line L7688 (174.3823, -3.418) -> (174.3823, -5.218)
  line L7689 (172.5823, -5.218) -> (172.5823, -3.418)
  line L7690 (174.3823, -5.218) -> (172.5823, -5.218)
  line L7691 (172.5823, -3.418) -> (174.3823, -3.418)
  line L7692 (172.5823, -3.418) -> (174.3823, -3.418)
  line L7693 (174.3823, -5.218) -> (172.5823, -5.218)
  line L7694 (174.3823, -3.418) -> (174.3823, -5.218)
  line L7695 (172.5823, -5.218) -> (172.5823, -3.418)
  arc A1784 (188.8893, -3.84) -> (188.2393, -3.84) centre (188.5643, -3.84) ccw
  arc A1785 (188.2393, -3.84) -> (188.8893, -3.84) centre (188.5643, -3.84) ccw
  arc A1786 (183.1092, -3.84) -> (182.4592, -3.84) centre (182.7842, -3.84) ccw
  arc A1787 (182.4592, -3.84) -> (183.1092, -3.84) centre (182.7842, -3.84) ccw
  arc A1788 (194.3974, -57.5184) -> (189.3974, -57.5184) centre (191.8974, -57.5184) ccw
  arc A1789 (189.3974, -57.5184) -> (194.3974, -57.5184) centre (191.8974, -57.5184) ccw
  arc A1790 (175.3474, -76.5812) -> (170.3473, -76.5812) centre (172.8473, -76.5812) ccw
  arc A1791 (170.3473, -76.5812) -> (175.3474, -76.5812) centre (172.8473, -76.5812) ccw
  arc A1792 (175.3474, -57.5184) -> (170.3473, -57.5184) centre (172.8473, -57.5184) ccw
  arc A1793 (170.3473, -57.5184) -> (175.3474, -57.5184) centre (172.8473, -57.5184) ccw
  arc A1794 (170.3473, -38.4557) -> (175.3474, -38.4557) centre (172.8473, -38.4557) ccw
  arc A1795 (175.3474, -38.4557) -> (170.3473, -38.4557) centre (172.8473, -38.4557) ccw
  arc A1796 (170.3473, -19.4056) -> (175.3474, -19.4056) centre (172.8473, -19.4056) ccw
  arc A1797 (175.3474, -19.4056) -> (170.3473, -19.4056) centre (172.8473, -19.4056) ccw
  arc A1798 (151.2973, -76.5812) -> (156.2973, -76.5812) centre (153.7973, -76.5812) ccw
  arc A1799 (156.2973, -76.5812) -> (151.2973, -76.5812) centre (153.7973, -76.5812) ccw
  arc A1800 (156.2973, -38.4557) -> (151.2973, -38.4557) centre (153.7973, -38.4557) ccw
  arc A1801 (151.2973, -38.4557) -> (156.2973, -38.4557) centre (153.7973, -38.4557) ccw
  arc A1802 (156.2973, -57.5184) -> (151.2973, -57.5184) centre (153.7973, -57.5184) ccw
  arc A1803 (151.2973, -57.5184) -> (156.2973, -57.5184) centre (153.7973, -57.5184) ccw
  arc A1804 (151.2973, -19.4056) -> (156.2973, -19.4056) centre (153.7973, -19.4056) ccw
  arc A1805 (156.2973, -19.4056) -> (151.2973, -19.4056) centre (153.7973, -19.4056) ccw
  arc A1806 (132.2473, -57.5184) -> (137.2473, -57.5184) centre (134.7473, -57.5184) ccw
  arc A1807 (137.2473, -57.5184) -> (132.2473, -57.5184) centre (134.7473, -57.5184) ccw
  arc A1808 (132.2473, -38.4557) -> (137.2473, -38.4557) centre (134.7473, -38.4557) ccw
  arc A1809 (137.2473, -38.4557) -> (132.2473, -38.4557) centre (134.7473, -38.4557) ccw
  arc A1810 (137.2473, -19.4056) -> (132.2473, -19.4056) centre (134.7473, -19.4056) ccw
  arc A1811 (132.2473, -19.4056) -> (137.2473, -19.4056) centre (134.7473, -19.4056) ccw
  arc A1812 (132.2473, -76.5812) -> (137.2473, -76.5812) centre (134.7473, -76.5812) ccw
  arc A1813 (137.2473, -76.5812) -> (132.2473, -76.5812) centre (134.7473, -76.5812) ccw
  arc A1814 (118.1972, -76.5812) -> (113.1972, -76.5812) centre (115.6972, -76.5812) ccw
  line L7696 (118.1972, -76.5812) -> (118.1972, -76.5812)
  arc A1815 (113.1972, -76.5812) -> (118.1972, -76.5812) centre (115.6972, -76.5812) ccw
  arc A1816 (113.1972, -57.5184) -> (118.1972, -57.5184) centre (115.6972, -57.5184) ccw
  arc A1817 (118.1972, -57.5184) -> (113.1972, -57.5184) centre (115.6972, -57.5184) ccw
  line L7697 (118.1972, -57.5184) -> (118.1972, -57.5184)
  arc A1818 (118.1972, -19.4056) -> (113.1972, -19.4056) centre (115.6972, -19.4056) ccw
  line L7698 (118.1972, -19.4056) -> (118.1972, -19.4056)
  arc A1819 (113.1972, -19.4056) -> (118.1972, -19.4056) centre (115.6972, -19.4056) ccw
  arc A1820 (118.1972, -38.4557) -> (113.1972, -38.4557) centre (115.6972, -38.4557) ccw
  line L7699 (118.1972, -38.4557) -> (118.1972, -38.4557)
  arc A1821 (113.1972, -38.4557) -> (118.1972, -38.4557) centre (115.6972, -38.4557) ccw
  arc A1822 (99.1472, -19.4056) -> (94.1472, -19.4056) centre (96.6472, -19.4056) ccw
  arc A1823 (94.1472, -19.4056) -> (99.1472, -19.4056) centre (96.6472, -19.4056) ccw
  line L7700 (99.1472, -19.4056) -> (99.1472, -19.4056)
  arc A1824 (94.1472, -38.4557) -> (99.1472, -38.4557) centre (96.6472, -38.4557) ccw
  arc A1825 (99.1472, -38.4557) -> (94.1472, -38.4557) centre (96.6472, -38.4557) ccw
  line L7701 (99.1472, -38.4557) -> (99.1472, -38.4557)
  line L7702 (99.1472, -76.5812) -> (99.1472, -76.5812)
  arc A1826 (99.1472, -76.5812) -> (94.1472, -76.5812) centre (96.6472, -76.5812) ccw
  arc A1827 (94.1472, -76.5812) -> (99.1472, -76.5812) centre (96.6472, -76.5812) ccw
  arc A1828 (94.1472, -57.5184) -> (99.1472, -57.5184) centre (96.6472, -57.5184) ccw
  arc A1829 (99.1472, -57.5184) -> (94.1472, -57.5184) centre (96.6472, -57.5184) ccw
  line L7703 (99.1472, -57.5184) -> (99.1472, -57.5184)
  arc A1830 (189.3974, -76.5812) -> (194.3974, -76.5812) centre (191.8974, -76.5812) ccw
  arc A1831 (194.3974, -76.5812) -> (189.3974, -76.5812) centre (191.8974, -76.5812) ccw
  arc A1832 (194.3974, -19.4056) -> (189.3974, -19.4056) centre (191.8974, -19.4056) ccw
  arc A1833 (189.3974, -19.4056) -> (194.3974, -19.4056) centre (191.8974, -19.4056) ccw
  arc A1834 (75.0972, -76.5812) -> (80.0972, -76.5812) centre (77.5972, -76.5812) ccw
  arc A1835 (80.0972, -76.5812) -> (75.0972, -76.5812) centre (77.5972, -76.5812) ccw
  line L7704 (80.0972, -76.5812) -> (80.0972, -76.5812)
  arc A1836 (80.0972, -38.4557) -> (75.0972, -38.4557) centre (77.5972, -38.4557) ccw
  line L7705 (80.0972, -38.4557) -> (80.0972, -38.4557)
  arc A1837 (75.0972, -38.4557) -> (80.0972, -38.4557) centre (77.5972, -38.4557) ccw
  line L7706 (80.0972, -19.4056) -> (80.0972, -19.4056)
  arc A1838 (75.0972, -19.4056) -> (80.0972, -19.4056) centre (77.5972, -19.4056) ccw
  arc A1839 (80.0972, -19.4056) -> (75.0972, -19.4056) centre (77.5972, -19.4056) ccw
  arc A1840 (80.0972, -57.5184) -> (75.0972, -57.5184) centre (77.5972, -57.5184) ccw
  arc A1841 (75.0972, -57.5184) -> (80.0972, -57.5184) centre (77.5972, -57.5184) ccw
  line L7707 (80.0972, -57.5184) -> (80.0972, -57.5184)
  arc A1842 (61.0471, -76.5812) -> (56.0471, -76.5812) centre (58.5471, -76.5812) ccw
  arc A1843 (56.0471, -76.5812) -> (61.0471, -76.5812) centre (58.5471, -76.5812) ccw
  arc A1844 (61.0471, -57.5184) -> (56.0471, -57.5184) centre (58.5471, -57.5184) ccw
  arc A1845 (56.0471, -57.5184) -> (61.0471, -57.5184) centre (58.5471, -57.5184) ccw
  arc A1846 (56.0471, -38.4557) -> (61.0471, -38.4557) centre (58.5471, -38.4557) ccw
  arc A1847 (61.0471, -38.4557) -> (56.0471, -38.4557) centre (58.5471, -38.4557) ccw
  arc A1848 (41.9971, -57.5184) -> (36.9971, -57.5184) centre (39.4971, -57.5184) ccw
  arc A1849 (36.9971, -57.5184) -> (41.9971, -57.5184) centre (39.4971, -57.5184) ccw
  arc A1850 (41.9971, -76.5812) -> (36.9971, -76.5812) centre (39.4971, -76.5812) ccw
  arc A1851 (36.9971, -76.5812) -> (41.9971, -76.5812) centre (39.4971, -76.5812) ccw
  arc A1852 (17.947, -76.5812) -> (22.947, -76.5812) centre (20.447, -76.5812) ccw
  arc A1853 (22.947, -76.5812) -> (17.947, -76.5812) centre (20.447, -76.5812) ccw
  arc A1854 (-1.103, -76.5812) -> (3.897, -76.5812) centre (1.397, -76.5812) ccw
  arc A1855 (3.897, -76.5812) -> (-1.103, -76.5812) centre (1.397, -76.5812) ccw
  arc A1856 (61.0471, -19.4056) -> (56.0471, -19.4056) centre (58.5471, -19.4056) ccw
  arc A1857 (56.0471, -19.4056) -> (61.0471, -19.4056) centre (58.5471, -19.4056) ccw
  arc A1858 (41.9971, -38.4557) -> (36.9971, -38.4557) centre (39.4971, -38.4557) ccw
  arc A1859 (36.9971, -38.4557) -> (41.9971, -38.4557) centre (39.4971, -38.4557) ccw
  arc A1860 (36.9971, -19.4056) -> (41.9971, -19.4056) centre (39.4971, -19.4056) ccw
  arc A1861 (41.9971, -19.4056) -> (36.9971, -19.4056) centre (39.4971, -19.4056) ccw
  arc A1862 (17.947, -19.4056) -> (22.947, -19.4056) centre (20.447, -19.4056) ccw
  arc A1863 (22.947, -19.4056) -> (17.947, -19.4056) centre (20.447, -19.4056) ccw
  arc A1864 (22.947, -57.5184) -> (17.947, -57.5184) centre (20.447, -57.5184) ccw
  arc A1865 (17.947, -57.5184) -> (22.947, -57.5184) centre (20.447, -57.5184) ccw
  arc A1866 (17.947, -38.4557) -> (22.947, -38.4557) centre (20.447, -38.4557) ccw
  arc A1867 (22.947, -38.4557) -> (17.947, -38.4557) centre (20.447, -38.4557) ccw
  arc A1868 (3.897, -19.4056) -> (-1.103, -19.4056) centre (1.397, -19.4056) ccw
  arc A1869 (-1.103, -19.4056) -> (3.897, -19.4056) centre (1.397, -19.4056) ccw
  arc A1870 (3.897, -38.4557) -> (-1.103, -38.4557) centre (1.397, -38.4557) ccw
  arc A1871 (-1.103, -38.4557) -> (3.897, -38.4557) centre (1.397, -38.4557) ccw
  arc A1872 (-1.103, -57.5184) -> (3.897, -57.5184) centre (1.397, -57.5184) ccw
  arc A1873 (3.897, -57.5184) -> (-1.103, -57.5184) centre (1.397, -57.5184) ccw
  arc A1874 (208.4474, -57.5184) -> (213.4474, -57.5184) centre (210.9474, -57.5184) ccw
  arc A1875 (213.4474, -57.5184) -> (208.4474, -57.5184) centre (210.9474, -57.5184) ccw
  arc A1876 (213.4474, -38.4557) -> (208.4474, -38.4557) centre (210.9474, -38.4557) ccw
  arc A1877 (208.4474, -38.4557) -> (213.4474, -38.4557) centre (210.9474, -38.4557) ccw
  arc A1878 (213.4474, -19.4056) -> (208.4474, -19.4056) centre (210.9474, -19.4056) ccw
  arc A1879 (208.4474, -19.4056) -> (213.4474, -19.4056) centre (210.9474, -19.4056) ccw
  arc A1880 (208.4474, -76.5812) -> (213.4474, -76.5812) centre (210.9474, -76.5812) ccw
  arc A1881 (213.4474, -76.5812) -> (208.4474, -76.5812) centre (210.9474, -76.5812) ccw
  arc A1882 (194.3974, -38.4557) -> (189.3974, -38.4557) centre (191.8974, -38.4557) ccw
  arc A1883 (189.3974, -38.4557) -> (194.3974, -38.4557) centre (191.8974, -38.4557) ccw
  arc A1884 (207.1995, -6.1629) -> (207.3494, -6.1629) centre (207.2744, -6.1629) ccw
  arc A1885 (207.3494, -6.1629) -> (207.1995, -6.1629) centre (207.2744, -6.1629) ccw
  arc A1886 (212.8031, -3.2765) -> (213.0033, -3.2765) centre (212.9032, -3.2765) ccw
  arc A1887 (213.0033, -3.2765) -> (212.8031, -3.2765) centre (212.9032, -3.2765) ccw
  arc A1888 (194.9835, -3.7496) -> (194.7833, -3.7496) centre (194.8834, -3.7496) ccw
  arc A1889 (194.7833, -3.7496) -> (194.9835, -3.7496) centre (194.8834, -3.7496) ccw
  line L7708 (139.549, -76.7538) -> (138.733, -76.7538)
  line L7709 (138.733, -76.7538) -> (138.733, -76.9578)
  line L7710 (139.549, -76.9578) -> (139.549, -76.7538)
  line L7711 (138.733, -76.9578) -> (139.549, -76.9578)
  line L7712 (141.5169, -77.5359) -> (141.5169, -76.1758)
  line L7713 (141.5169, -76.1758) -> (141.7209, -76.1758)
  line L7714 (141.7209, -76.1758) -> (141.7209, -77.5359)
  line L7715 (141.7209, -77.5359) -> (141.5169, -77.5359)
  line L7716 (142.0269, -76.9579) -> (141.2109, -76.9579)
  line L7717 (142.0269, -76.7538) -> (142.0269, -76.9579)
  line L7718 (141.2109, -76.7538) -> (142.0269, -76.7538)
  line L7719 (141.2109, -76.9579) -> (141.2109, -76.7538)
  line L7720 (138.733, -19.5783) -> (138.733, -19.7823)
  line L7721 (139.549, -19.7823) -> (139.549, -19.5783)
  line L7722 (139.549, -19.5783) -> (138.733, -19.5783)
  line L7723 (138.733, -19.7823) -> (139.549, -19.7823)
  line L7724 (141.5169, -20.3604) -> (141.5169, -19.0003)
  line L7725 (141.7209, -20.3604) -> (141.5169, -20.3604)
  line L7726 (141.7209, -19.0003) -> (141.7209, -20.3604)
  line L7727 (141.5169, -19.0003) -> (141.7209, -19.0003)
  line L7728 (142.0269, -19.5783) -> (142.0269, -19.7823)
  line L7729 (141.2109, -19.7823) -> (141.2109, -19.5783)
  line L7730 (142.0269, -19.7823) -> (141.2109, -19.7823)
  line L7731 (141.2109, -19.5783) -> (142.0269, -19.5783)
  line L7732 (138.733, -38.6283) -> (138.733, -38.8324)
  line L7733 (139.549, -38.8324) -> (139.549, -38.6283)
  line L7734 (139.549, -38.6283) -> (138.733, -38.6283)
  line L7735 (138.733, -38.8324) -> (139.549, -38.8324)
  line L7736 (141.7209, -39.4104) -> (141.5169, -39.4104)
  line L7737 (141.7209, -38.0504) -> (141.7209, -39.4104)
  line L7738 (141.5169, -39.4104) -> (141.5169, -38.0504)
  line L7739 (141.5169, -38.0504) -> (141.7209, -38.0504)
  line L7740 (141.2109, -38.6284) -> (142.0269, -38.6284)
  line L7741 (141.2109, -38.8324) -> (141.2109, -38.6284)
  line L7742 (142.0269, -38.6284) -> (142.0269, -38.8324)
  line L7743 (142.0269, -38.8324) -> (141.2109, -38.8324)
  line L7744 (139.549, -57.8951) -> (139.549, -57.6911)
  line L7745 (138.733, -57.8951) -> (139.549, -57.8951)
  line L7746 (139.549, -57.6911) -> (138.733, -57.6911)
  line L7747 (138.733, -57.6911) -> (138.733, -57.8951)
  line L7748 (141.7209, -58.4731) -> (141.5169, -58.4731)
  line L7749 (141.5169, -57.1131) -> (141.7209, -57.1131)
  line L7750 (141.5169, -58.4731) -> (141.5169, -57.1131)
  line L7751 (141.7209, -57.1131) -> (141.7209, -58.4731)
  line L7752 (142.0269, -57.8951) -> (141.2109, -57.8951)
  line L7753 (142.0269, -57.6911) -> (142.0269, -57.8951)
  line L7754 (141.2109, -57.8951) -> (141.2109, -57.6911)
  line L7755 (141.2109, -57.6911) -> (142.0269, -57.6911)
  line L7756 (158.5991, -19.7823) -> (158.5991, -19.5783)
  line L7757 (157.7831, -19.5783) -> (157.7831, -19.7823)
  line L7758 (157.7831, -19.7823) -> (158.5991, -19.7823)
  line L7759 (158.5991, -19.5783) -> (157.7831, -19.5783)
  line L7760 (160.5669, -20.3604) -> (160.5669, -19.0003)
  line L7761 (160.7709, -19.0003) -> (160.7709, -20.3604)
  line L7762 (160.7709, -20.3604) -> (160.5669, -20.3604)
  line L7763 (160.5669, -19.0003) -> (160.7709, -19.0003)
  line L7764 (160.2609, -19.7823) -> (160.2609, -19.5783)
  line L7765 (161.0769, -19.7823) -> (160.2609, -19.7823)
  line L7766 (161.0769, -19.5783) -> (161.0769, -19.7823)
  line L7767 (160.2609, -19.5783) -> (161.0769, -19.5783)
  line L7768 (157.7831, -76.9578) -> (158.5991, -76.9578)
  line L7769 (157.7831, -76.7538) -> (157.7831, -76.9578)
  line L7770 (158.5991, -76.7538) -> (157.7831, -76.7538)
  line L7771 (158.5991, -76.9578) -> (158.5991, -76.7538)
  line L7772 (160.7709, -76.1758) -> (160.7709, -77.5359)
  line L7773 (160.5669, -77.5359) -> (160.5669, -76.1758)
  line L7774 (160.7709, -77.5359) -> (160.5669, -77.5359)
  line L7775 (160.5669, -76.1758) -> (160.7709, -76.1758)
  line L7776 (160.2609, -76.9579) -> (160.2609, -76.7538)
  line L7777 (161.0769, -76.7538) -> (161.0769, -76.9579)
  line L7778 (161.0769, -76.9579) -> (160.2609, -76.9579)
  line L7779 (160.2609, -76.7538) -> (161.0769, -76.7538)
  line L7780 (158.5991, -57.6911) -> (157.7831, -57.6911)
  line L7781 (158.5991, -57.8951) -> (158.5991, -57.6911)
  line L7782 (157.7831, -57.6911) -> (157.7831, -57.8951)
  line L7783 (157.7831, -57.8951) -> (158.5991, -57.8951)
  line L7784 (160.7709, -57.1131) -> (160.7709, -58.4731)
  line L7785 (160.5669, -58.4731) -> (160.5669, -57.1131)
  line L7786 (160.7709, -58.4731) -> (160.5669, -58.4731)
  line L7787 (160.5669, -57.1131) -> (160.7709, -57.1131)
  line L7788 (160.2609, -57.6911) -> (161.0769, -57.6911)
  line L7789 (161.0769, -57.6911) -> (161.0769, -57.8951)
  line L7790 (161.0769, -57.8951) -> (160.2609, -57.8951)
  line L7791 (160.2609, -57.8951) -> (160.2609, -57.6911)
  line L7792 (158.5991, -38.6283) -> (157.7831, -38.6283)
  line L7793 (157.7831, -38.6283) -> (157.7831, -38.8324)
  line L7794 (157.7831, -38.8324) -> (158.5991, -38.8324)
  line L7795 (158.5991, -38.8324) -> (158.5991, -38.6283)
  line L7796 (160.7709, -39.4104) -> (160.5669, -39.4104)
  line L7797 (160.7709, -38.0504) -> (160.7709, -39.4104)
  line L7798 (160.5669, -38.0504) -> (160.7709, -38.0504)
  line L7799 (160.5669, -39.4104) -> (160.5669, -38.0504)
  line L7800 (161.0769, -38.6284) -> (161.0769, -38.8324)
  line L7801 (161.0769, -38.8324) -> (160.2609, -38.8324)
  line L7802 (160.2609, -38.6284) -> (161.0769, -38.6284)
  line L7803 (160.2609, -38.8324) -> (160.2609, -38.6284)
  line L7804 (177.6491, -19.7823) -> (177.6491, -19.5783)
  line L7805 (177.6491, -19.5783) -> (176.8331, -19.5783)
  line L7806 (176.8331, -19.5783) -> (176.8331, -19.7823)
  line L7807 (176.8331, -19.7823) -> (177.6491, -19.7823)
  line L7808 (179.821, -20.3604) -> (179.617, -20.3604)
  line L7809 (179.617, -20.3604) -> (179.617, -19.0003)
  line L7810 (179.821, -19.0003) -> (179.821, -20.3604)
  line L7811 (179.617, -19.0003) -> (179.821, -19.0003)
  line L7812 (179.311, -19.7823) -> (179.311, -19.5783)